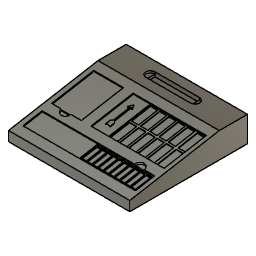
mme_projekt (Autodesk Fusion 360 design; units mm, degrees)
Autodesk Fusion 360 part; units mm, degrees
note: some values were not read from the file. Set by a fixed rule: which sketch regions a step uses.
sketch "Base" plane through (0, 0, 0) normal (1, 0, 0) x (0, 1, 0)
  line L0 (0, 0) -> (0, 20)
  line L1 (0, 20) -> (184.2, 20)
  line L2 (184.2, 20) -> (184.2, 0)
  line L3 (184.2, 0) -> (0, 0)
  line L4 (184.2, 20) -> (184.2, 52.4794)
  line L5 (184.2, 52.4794) -> (0, 20)
  line L6 (184.2, 52.4794) -> (242.2, 52.4794)
  line L7 (242.2, 52.4794) -> (242.2, 0)
  line L8 (242.2, 0) -> (184.2, 0)
  dimension "d6" = 10
  dimension "d7" = 58
  dimension "d8" = 184.2
  dimension "d9" = 20
  constraint coincident L0.start L3.end
  constraint vertical L0
  constraint perpendicular L0 L1
  constraint perpendicular L1 L2
  constraint perpendicular L0 L3
  constraint perpendicular L1 L4
  constraint perpendicular L0 L6
  constraint perpendicular L1 L7
  constraint perpendicular L2 L8
  measures "d6" angle of L1 L5
  measures "d7" distance of L2.end L7.end
  measures "d8" distance of L2.end L0.start
  measures "d9" distance of L0.start L0.end
sketch "Main Indents" plane through (0, -3.4202, 19.3969) normal (0, -0.173648, 0.984808) x (1, 0, 0)
  line L0 (0, 190.5145) -> (0, 3.473)
  line L1 (0, 3.473) -> (10, 3.473)
  line L2 (10, 3.473) -> (10, 190.5145)
  line L3 (10, 190.5145) -> (0, 190.5145)
  line L4 (8, 83.473) -> (71, 83.473)
  line L5 (71, 83.473) -> (71, 171.473)
  line L6 (71, 171.473) -> (8, 171.473)
  line L7 (8, 171.473) -> (8, 83.473)
  line L8 (181, 129.5926) -> (166, 129.5926)
  line L9 (166, 169.5926) -> (166, 129.5926)
  line L10 (166, 169.5926) -> (181, 169.5926)
  line L11 (181, 169.5926) -> (181, 129.5926)
  line L12 (147, 169.5926) -> (162, 169.5926)
  line L13 (162, 169.5926) -> (162, 129.5926)
  line L14 (128, 169.5926) -> (128, 129.5926)
  line L15 (143, 129.5926) -> (128, 129.5926)
  line L16 (147, 169.5926) -> (147, 129.5926)
  line L17 (128, 169.5926) -> (143, 169.5926)
  line L18 (143, 169.5926) -> (143, 129.5926)
  line L19 (162, 129.5926) -> (147, 129.5926)
  line L20 (162, 125.5926) -> (162, 85.5926)
  line L21 (128, 125.5926) -> (143, 125.5926)
  line L22 (166, 125.5926) -> (166, 85.5926)
  line L23 (181, 85.5926) -> (166, 85.5926)
  line L24 (166, 125.5926) -> (181, 125.5926)
  line L25 (147, 125.5926) -> (162, 125.5926)
  line L26 (128, 125.5926) -> (128, 85.5926)
  line L27 (162, 85.5926) -> (147, 85.5926)
  line L28 (147, 125.5926) -> (147, 85.5926)
  line L29 (143, 125.5926) -> (143, 85.5926)
  line L30 (143, 85.5926) -> (128, 85.5926)
  line L31 (181, 125.5926) -> (181, 85.5926)
  line L32 (143, 129.5926) -> (147, 129.5926) construction
  line L33 (162, 129.5926) -> (166, 129.5926) construction
  line L34 (166, 125.5926) -> (162, 125.5926) construction
  line L35 (147, 125.5926) -> (143, 125.5926) construction
  line L36 (185, 169.5926) -> (200, 169.5926)
  line L37 (200, 169.5926) -> (200, 129.5926)
  line L38 (185, 169.5926) -> (185, 129.5926)
  line L39 (200, 129.5926) -> (185, 129.5926)
  line L40 (204, 169.5926) -> (219, 169.5926)
  line L41 (219, 169.5926) -> (219, 129.5926)
  line L42 (204, 169.5926) -> (204, 129.5926)
  line L43 (219, 129.5926) -> (204, 129.5926)
  line L44 (224.5079, 169.5926) -> (239.5079, 169.5926)
  line L45 (239.5079, 169.5926) -> (239.5079, 129.5926)
  line L46 (224.5079, 169.5926) -> (224.5079, 129.5926)
  line L47 (239.5079, 129.5926) -> (224.5079, 129.5926)
  line L48 (185, 125.5926) -> (200, 125.5926)
  line L49 (200, 125.5926) -> (200, 85.5926)
  line L50 (185, 125.5926) -> (185, 85.5926)
  line L51 (200, 85.5926) -> (185, 85.5926)
  line L52 (204, 125.5926) -> (219, 125.5926)
  line L53 (219, 125.5926) -> (219, 85.5926)
  line L54 (204, 125.5926) -> (204, 85.5926)
  line L55 (219, 85.5926) -> (204, 85.5926)
  line L56 (224.5079, 125.5926) -> (239.5079, 125.5926)
  line L57 (239.5079, 125.5926) -> (239.5079, 85.5926)
  line L58 (224.5079, 125.5926) -> (224.5079, 85.5926)
  line L59 (239.5079, 85.5926) -> (224.5079, 85.5926)
  line L60 (185, 129.5926) -> (185, 125.5926) construction
  line L61 (185, 125.5926) -> (181, 125.5926) construction
  line L62 (181, 129.5926) -> (185, 129.5926) construction
  line L63 (204, 129.5926) -> (200, 129.5926) construction
  line L64 (200, 125.5926) -> (204, 125.5926) construction
  line L65 (204, 125.5926) -> (204, 129.5926) construction
  line L66 (224.5079, 125.5926) -> (224.5079, 129.5926) construction
  line L67 (219, 129.5926) -> (224.5079, 129.5926) construction
  line L68 (224.5079, 125.5926) -> (219, 125.5926) construction
  line L69 (91, 171.473) -> (241.5079, 171.473)
  line L70 (241.5079, 171.473) -> (241.5079, 83.473)
  line L71 (241.5079, 83.473) -> (91, 83.473)
  line L72 (91, 83.473) -> (91, 171.473)
  line L73 (71, 171.473) -> (91, 171.473) construction
  line L74 (8, 63.473) -> (241.5079, 63.473)
  line L75 (241.5079, 63.473) -> (241.5079, 23.473)
  line L76 (241.5079, 23.473) -> (8, 23.473)
  line L77 (8, 23.473) -> (8, 63.473)
  line L78 (8, 83.473) -> (8, 63.473) construction
  line L79 (71, 83.473) -> (91, 83.473) construction
  line L80 (216.5079, 58.973) -> (216.5079, 27.973)
  line L81 (225.7579, 27.973) -> (225.7579, 58.973)
  line L82 (225.7579, 58.973) -> (216.5079, 58.973)
  line L83 (216.5079, 27.973) -> (225.7579, 27.973)
  line L84 (205.2579, 58.973) -> (205.2579, 27.973)
  line L85 (214.5079, 27.973) -> (214.5079, 58.973)
  line L86 (214.5079, 58.973) -> (205.2579, 58.973)
  line L87 (205.2579, 27.973) -> (214.5079, 27.973)
  line L88 (194.0079, 58.973) -> (194.0079, 27.973)
  line L89 (203.2579, 27.973) -> (203.2579, 58.973)
  line L90 (203.2579, 58.973) -> (194.0079, 58.973)
  line L91 (194.0079, 27.973) -> (203.2579, 27.973)
  line L92 (227.7579, 58.973) -> (227.7579, 27.973)
  line L93 (237.0079, 27.973) -> (237.0079, 58.973)
  line L94 (237.0079, 58.973) -> (227.7579, 58.973)
  line L95 (227.7579, 27.973) -> (237.0079, 27.973)
  line L96 (182.7579, 58.973) -> (182.7579, 27.973)
  line L97 (192.0079, 27.973) -> (192.0079, 58.973)
  line L98 (192.0079, 58.973) -> (182.7579, 58.973)
  line L99 (182.7579, 27.973) -> (192.0079, 27.973)
  line L100 (171.5079, 58.973) -> (171.5079, 27.973)
  line L101 (180.7579, 27.973) -> (180.7579, 58.973)
  line L102 (180.7579, 58.973) -> (171.5079, 58.973)
  line L103 (171.5079, 27.973) -> (180.7579, 27.973)
  line L104 (160.2579, 58.973) -> (160.2579, 27.973)
  line L105 (169.5079, 27.973) -> (169.5079, 58.973)
  line L106 (169.5079, 58.973) -> (160.2579, 58.973)
  line L107 (160.2579, 27.973) -> (169.5079, 27.973)
  line L108 (149.0079, 58.973) -> (149.0079, 27.973)
  line L109 (158.2579, 27.973) -> (158.2579, 58.973)
  line L110 (158.2579, 58.973) -> (149.0079, 58.973)
  line L111 (149.0079, 27.973) -> (158.2579, 27.973)
  line L112 (137.7579, 58.973) -> (137.7579, 27.973)
  line L113 (147.0079, 27.973) -> (147.0079, 58.973)
  line L114 (147.0079, 58.973) -> (137.7579, 58.973)
  line L115 (137.7579, 27.973) -> (147.0079, 27.973)
  line L116 (126.5079, 58.973) -> (126.5079, 27.973)
  line L117 (135.7579, 27.973) -> (135.7579, 58.973)
  line L118 (135.7579, 58.973) -> (126.5079, 58.973)
  line L119 (126.5079, 27.973) -> (135.7579, 27.973)
  line L120 (227.7579, 58.973) -> (225.7579, 58.973) construction
  line L121 (216.5079, 58.973) -> (214.5079, 58.973) construction
  line L122 (205.2579, 58.973) -> (203.2579, 58.973) construction
  line L123 (194.0079, 58.973) -> (192.0079, 58.973) construction
  line L124 (182.7579, 58.973) -> (180.7579, 58.973) construction
  line L125 (171.5079, 58.973) -> (169.5079, 58.973) construction
  line L126 (160.2579, 58.973) -> (158.2579, 58.973) construction
  line L127 (149.0079, 58.973) -> (147.0079, 58.973) construction
  line L128 (137.7579, 58.973) -> (135.7579, 58.973) construction
  line L129 (216.5079, 27.973) -> (214.5079, 27.973) construction
  line L130 (205.2579, 27.973) -> (203.2579, 27.973) construction
  line L131 (194.0079, 27.973) -> (192.0079, 27.973) construction
  line L132 (182.7579, 27.973) -> (180.7579, 27.973) construction
  line L133 (171.5079, 27.973) -> (169.5079, 27.973) construction
  line L134 (160.2579, 27.973) -> (158.2579, 27.973) construction
  line L135 (149.0079, 27.973) -> (147.0079, 27.973) construction
  line L136 (137.7579, 27.973) -> (135.7579, 27.973) construction
  line L137 (227.7579, 27.973) -> (225.7579, 27.973) construction
  line L138 (124.5079, 60.973) -> (124.5079, 25.973)
  line L139 (239.0079, 60.973) -> (239.0079, 25.973)
  line L140 (237.0079, 58.973) -> (239.0079, 58.973) construction
  line L141 (237.0079, 27.973) -> (239.0079, 27.973) construction
  line L142 (126.5079, 58.973) -> (124.5079, 58.973) construction
  line L143 (126.5079, 27.973) -> (124.5079, 27.973) construction
  line L144 (241.5079, 83.473) -> (241.5079, 63.473) construction
  line L145 (126, 171.473) -> (126, 83.473)
  line L146 (128, 129.5926) -> (128, 125.5926) construction
  line L147 (124.5079, 60.973) -> (239.0079, 60.973)
  line L148 (239.0079, 25.973) -> (124.5079, 25.973)
  arc A0 (29.5, 83.473) -> (49.5, 83.473) centre (39.5, 83.473) ccw
  line L149 (39.5, 171.473) -> (39.5, 83.473)
  line L150 (8, 43.473) -> (241.5079, 43.473)
  line L151 (107.5, 113.6221) -> (107.5, 148.6221)
  line L152 (107.5, 148.6221) -> (103.5, 146.3127)
  line L153 (103.5, 146.3127) -> (108.5, 154.973)
  line L154 (108.5, 154.973) -> (113.5, 146.3127)
  line L155 (113.5, 146.3127) -> (109.5, 148.6221)
  line L156 (109.5, 148.6221) -> (109.5, 113.6221)
  line L157 (109.5, 113.6221) -> (113.0355, 110.0866)
  line L158 (113.0355, 110.0866) -> (113.0355, 100.0866)
  line L159 (113.0355, 100.0866) -> (109.5, 102.1624)
  line L160 (109.5, 102.1624) -> (107.5, 102.1624)
  line L161 (107.5, 102.1624) -> (103.9645, 99.973)
  line L162 (103.9645, 99.973) -> (103.9645, 110.0866)
  line L163 (103.9645, 110.0866) -> (107.5, 113.6221)
  line L164 (107.5, 148.6221) -> (109.5, 148.6221) construction
  line L165 (107.5, 113.6221) -> (107.5, 102.1624) construction
  line L166 (109.5, 113.6221) -> (109.5, 102.1624) construction
  line L167 (107.5, 113.6221) -> (109.5, 113.6221) construction
  line L168 (103.9645, 99.973) -> (103.9645, 83.473) construction
  line L169 (108.5, 154.973) -> (108.5, 171.473) construction
  line L170 (126, 154.973) -> (91, 154.973) construction
  arc A1 (220.0079, 63.473) -> (200.0079, 63.473) centre (210.0079, 63.473) ccw
  dimension "d12" = 88
  dimension "d13" = 63
  dimension "d16" = 40
  dimension "d17" = 15
  dimension "d18" = 40
  dimension "d19" = 15
  dimension "d20" = 40
  dimension "d21" = 15
  dimension "d24" = 40
  dimension "d25" = 15
  dimension "d26" = 40
  dimension "d27" = 15
  dimension "d28" = 40
  dimension "d29" = 15
  dimension "d31" = 4
  dimension "d32" = 4
  dimension "d33" = 4
  dimension "d34" = 4
  dimension "d44" = 40
  dimension "d45" = 15
  dimension "d46" = 40
  dimension "d47" = 15
  dimension "d48" = 40
  dimension "d49" = 15
  dimension "d52" = 40
  dimension "d53" = 15
  dimension "d54" = 40
  dimension "d55" = 15
  dimension "d56" = 40
  dimension "d57" = 15
  dimension "d58" = 4
  dimension "d59" = 4
  dimension "d60" = 5.5079
  dimension "d62" = 20
  dimension "d64" = 2
  dimension "d65" = 40
  dimension "d66" = 20
  dimension "d67" = 8
  dimension "d68" = 20
  dimension "d70" = 9.25
  dimension "d71" = 9.25
  dimension "d72" = 9.25
  dimension "d73" = 9.25
  dimension "d74" = 9.25
  dimension "d75" = 9.25
  dimension "d76" = 9.25
  dimension "d77" = 9.25
  dimension "d78" = 9.25
  dimension "d79" = 9.25
  dimension "d80" = 2
  dimension "d81" = 2
  dimension "d82" = 2
  dimension "d83" = 2
  dimension "d84" = 2
  dimension "d85" = 2
  dimension "d86" = 2
  dimension "d87" = 2
  dimension "d88" = 2
  dimension "d89" = 2
  dimension "d90" = 2
  dimension "d91" = 2
  dimension "d92" = 35
  dimension "d93" = 4
  dimension "d94" = 1.8804
  dimension "d95" = 2
  dimension "d96" = 2
  dimension "d97" = 2.5
  dimension "d98" = 2.5
  dimension "d99" = 2.5
  dimension "d100" = 10
  dimension "d136" = 60
  dimension "d137" = 60
  dimension "d138" = 10
  dimension "d139" = 10
  dimension "d140" = 135
  dimension "d141" = 135
  dimension "d142" = 5
  dimension "d143" = 5
  dimension "d144" = 10
  dimension "d146" = 2
  dimension "d147" = 16.5
  dimension "d148" = 16.5
  dimension "d149" = 35
  dimension "d202" = 10
  dimension "d203" = 21.5
  constraint horizontal L4
  constraint perpendicular L4 L5
  constraint perpendicular L5 L6
  constraint perpendicular L4 L7
  constraint vertical L9
  constraint perpendicular L9 L10
  constraint perpendicular L10 L11
  constraint perpendicular L8 L9
  constraint vertical L16
  constraint perpendicular L12 L16
  constraint perpendicular L12 L13
  constraint perpendicular L16 L19
  constraint vertical L14
  constraint perpendicular L14 L17
  constraint perpendicular L17 L18
  constraint perpendicular L14 L15
  constraint vertical L22
  constraint perpendicular L22 L24
  constraint perpendicular L24 L31
  constraint perpendicular L22 L23
  constraint vertical L26
  constraint perpendicular L21 L26
  constraint perpendicular L21 L29
  constraint perpendicular L26 L30
  constraint vertical L28
  constraint perpendicular L25 L28
  constraint perpendicular L20 L25
  constraint perpendicular L27 L28
  constraint perpendicular L18 L32
  constraint perpendicular L9 L33
  constraint vertical L38
  constraint perpendicular L36 L38
  constraint perpendicular L36 L37
  constraint perpendicular L38 L39
  constraint vertical L42
  constraint perpendicular L40 L42
  constraint perpendicular L40 L41
  constraint perpendicular L42 L43
  constraint vertical L46
  constraint perpendicular L44 L46
  constraint perpendicular L44 L45
  constraint perpendicular L46 L47
  constraint vertical L50
  constraint perpendicular L48 L50
  constraint perpendicular L48 L49
  constraint perpendicular L50 L51
  constraint vertical L54
  constraint perpendicular L52 L54
  constraint perpendicular L52 L53
  constraint perpendicular L54 L55
  constraint vertical L58
  constraint perpendicular L56 L58
  constraint perpendicular L56 L57
  constraint perpendicular L58 L59
  constraint perpendicular L38 L62
  constraint perpendicular L37 L63
  constraint perpendicular L49 L64
  constraint perpendicular L63 L65
  constraint perpendicular L46 L67
  constraint perpendicular L53 L68
  constraint perpendicular L31 L61
  constraint perpendicular L47 L66
  constraint perpendicular L69 L70
  constraint perpendicular L5 L71
  constraint perpendicular L72 L73
  constraint parallel L4 L74
  constraint perpendicular L4 L75
  constraint perpendicular L2 L76
  constraint perpendicular L74 L77
  constraint perpendicular L74 L78
  constraint perpendicular L72 L79
  constraint horizontal L82
  constraint vertical L80
  constraint horizontal L83
  constraint vertical L81
  constraint horizontal L86
  constraint vertical L84
  constraint horizontal L87
  constraint vertical L85
  constraint horizontal L90
  constraint vertical L88
  constraint horizontal L91
  constraint vertical L89
  constraint horizontal L94
  constraint vertical L92
  constraint horizontal L95
  constraint vertical L93
  constraint horizontal L98
  constraint vertical L96
  constraint horizontal L99
  constraint vertical L97
  constraint horizontal L102
  constraint vertical L100
  constraint horizontal L103
  constraint vertical L101
  constraint horizontal L106
  constraint vertical L104
  constraint horizontal L107
  constraint vertical L105
  constraint horizontal L110
  constraint vertical L108
  constraint horizontal L111
  constraint vertical L109
  constraint horizontal L114
  constraint vertical L112
  constraint horizontal L115
  constraint vertical L113
  constraint horizontal L118
  constraint vertical L116
  constraint horizontal L119
  constraint vertical L117
  constraint perpendicular L81 L120
  constraint perpendicular L85 L121
  constraint perpendicular L89 L122
  constraint perpendicular L97 L123
  constraint perpendicular L101 L124
  constraint perpendicular L105 L125
  constraint perpendicular L104 L126
  constraint perpendicular L113 L127
  constraint perpendicular L117 L128
  constraint perpendicular L85 L129
  constraint perpendicular L89 L130
  constraint perpendicular L96 L132
  constraint perpendicular L105 L133
  constraint perpendicular L113 L135
  constraint perpendicular L117 L136
  constraint perpendicular L109 L134
  constraint perpendicular L88 L131
  constraint perpendicular L81 L137
  constraint vertical L138
  constraint vertical L139
  constraint coincident L139 L140.end
  constraint perpendicular L139 L140
  constraint coincident L139 L141.end
  constraint perpendicular L139 L141
  constraint coincident L138 L142.end
  constraint perpendicular L138 L142
  constraint coincident L138 L143.end
  constraint perpendicular L138 L143
  constraint perpendicular L20 L34
  constraint perpendicular L28 L35
  constraint perpendicular L74 L144
  constraint coincident L69 L145.start
  constraint coincident L71 L145.end
  constraint perpendicular L71 L145
  constraint perpendicular L39 L60
  constraint perpendicular L21 L146
  constraint perpendicular L138 L148
  constraint perpendicular L139 L147
  constraint coincident L4 A0.start
  constraint coincident L4 A0.centre
  constraint midpoint L6 L149.start
  constraint midpoint L4 A0.centre
  constraint coincident A0.centre L149
  constraint coincident L77 L150.start
  constraint midpoint L75 L150.end
  constraint midpoint L77 L150.start
  constraint vertical L151
  constraint perpendicular L152 L154
  constraint perpendicular L153 L155
  constraint vertical L156
  constraint parallel L156 L158
  constraint perpendicular L158 L160
  constraint perpendicular L160 L162
  constraint perpendicular L151 L164
  constraint parallel L151 L165
  constraint parallel L156 L166
  constraint perpendicular L151 L167
  constraint coincident L71 L168.end
  constraint perpendicular L71 L168
  constraint coincident L69 L169.end
  constraint perpendicular L69 L169
  constraint coincident L145 L170.start
  constraint coincident L72 L170.end
  constraint perpendicular L72 L170
  constraint midpoint L153.end L170
  constraint coincident L74 A1.start
  constraint coincident L74 A1.centre
  measures "d12" distance of L4.end L5.end
  measures "d13" distance of L4.start L4.end
  measures "d16" distance of L9.start L8.end
  measures "d17" distance of L9.start L10.end
  measures "d18" distance of L12.start L16.end
  measures "d19" distance of L12.start L12.end
  measures "d20" distance of L14.end L14.start
  measures "d21" distance of L17.end L14.start
  measures "d24" distance of L22.end L22.start
  measures "d25" distance of L24.end L22.start
  measures "d26" distance of L21.start L26.end
  measures "d27" distance of L21.start L21.end
  measures "d28" distance of L27.end L25.start
  measures "d29" distance of L20.start L25.start
  measures "d31" distance of L16 L18
  measures "d32" distance of L9 L13
  measures "d33" distance of L20 L22
  measures "d34" distance of L28 L29
  measures "d44" distance of L36.start L38.end
  measures "d45" distance of L36.start L36.end
  measures "d46" distance of L40.start L42.end
  measures "d47" distance of L40.start L40.end
  measures "d48" distance of L44.start L46.end
  measures "d49" distance of L44.start L44.end
  measures "d52" distance of L48.start L50.end
  measures "d53" distance of L48.start L48.end
  measures "d54" distance of L52.start L54.end
  measures "d55" distance of L52.start L52.end
  measures "d56" distance of L56.start L58.end
  measures "d57" distance of L56.start L56.end
  measures "d58" distance of L31 L50
  measures "d59" distance of L49 L54
  measures "d60" distance of L53 L58
  measures "d62" distance of L5 L72
  measures "d64" distance of L45 L70
  measures "d65" distance of L74.end L75.end
  measures "d66" distance of L1 L76
  measures "d67" distance of L0 L77
  measures "d68" distance of L4.start L74.start
  measures "d70" distance of L93.end L92.start
  measures "d71" distance of L81.end L80.start
  measures "d72" distance of L85.end L84.start
  measures "d73" distance of L89.end L88.start
  measures "d74" distance of L97.end L96.start
  measures "d75" distance of L101.end L100.start
  measures "d76" distance of L105.end L104.start
  measures "d77" distance of L109.end L108.start
  measures "d78" distance of L113.end L112.start
  measures "d79" distance of L117.end L116.start
  measures "d80" distance of L93.end L140.end
  measures "d81" distance of L81.end L92.start
  measures "d82" distance of L80.start L85.end
  measures "d83" distance of L84.start L89.end
  measures "d84" distance of L88.start L97.end
  measures "d85" distance of L96.start L101.end
  measures "d86" distance of L100.start L105.end
  measures "d87" distance of L104.start L109.end
  measures "d88" distance of L108.start L113.end
  measures "d89" distance of L112.start L117.end
  measures "d90" distance of L116.start L142.end
  measures "d91" distance of L14 L145
  measures "d92" distance of L72 L145.start
  measures "d93" distance of L15 L21
  measures "d94" distance of L17 L69
  measures "d95" distance of L118 L147
  measures "d96" distance of L119 L148
  measures "d97" distance of L76 L148
  measures "d98" distance of L74 L147
  measures "d99" distance of L75 L139
  measures "d100" radius of A0
  measures "d136" angle of L151 L152
  measures "d137" angle of L155 L156
  measures "d138" distance of L152.end L153.end
  measures "d139" distance of L153.end L154.end
  measures "d140" angle of L151 L163
  measures "d141" angle of L156 L157
  measures "d142" distance of L156.end L157.end
  measures "d143" distance of L151.start L162.end
  measures "d144" distance of L157.end L158.end
  measures "d146" distance of L159.end L160.end
  measures "d147" distance of L153.end L169.end
  measures "d148" distance of L161.end L168.end
  measures "d149" distance of L151.start L151.end
  measures "d202" radius of A1
  measures "d203" distance of L74.end A1.start
extrude "Extrude16" add sketch "Base" along normal blind 249.5
sketch "Top Indents" plane through (0, 0, 52.4794) normal (0, 0, 1) x (-1, 0, 0)
  line L0 (0, -242.2) -> (0, -184.2)
  line L1 (0, -184.2) -> (-249.5, -184.2)
  line L2 (-249.5, -184.2) -> (-249.5, -242.2)
  line L3 (-249.5, -242.2) -> (0, -242.2)
  line L4 (-78.75, -222.7) -> (-78.75, -203.7)
  line L5 (-78.75, -222.7) -> (-170.75, -222.7)
  line L6 (-170.75, -222.7) -> (-170.75, -203.7)
  line L7 (-170.75, -203.7) -> (-78.75, -203.7)
  line L8 (-124.75, -222.7) -> (-124.75, -203.7)
  line L9 (-249.5, -213.2) -> (0, -213.2)
  line L10 (-124.75, -242.2) -> (-124.75, -184.2)
  arc A0 (-170.75, -203.7) -> (-170.75, -222.7) centre (-170.75, -213.2) ccw
  arc A1 (-78.75, -222.7) -> (-78.75, -203.7) centre (-78.75, -213.2) ccw
  dimension "d210" = 19
  dimension "d211" = 92
  constraint perpendicular L3 L4
  constraint perpendicular L4 L5
  constraint perpendicular L5 L6
  constraint perpendicular L6 L7
  constraint midpoint L5 L8.start
  constraint midpoint L7 L8.end
  constraint midpoint L2 L9.start
  constraint midpoint L0 L9.end
  constraint midpoint L3 L10.start
  constraint midpoint L1 L10.end
  constraint midpoint L8 L10
  constraint midpoint L6 A0.centre
  constraint midpoint L4 A1.centre
  measures "d210" distance of L4.start L4.end
  measures "d211" distance of L4.start L5.end
extrude "Extrude17" cut sketch "Top Indents" against normal blind 9 contours L4 L5 L8 L9 L10 | L5 L6 L8 L9 L10 | L4 L7 L8 L9 L10 | L6 L7 L8 L9 L10
extrude "Extrude18" cut sketch "Top Indents" against normal blind 4 contours L4 L9 A1 | L4 L9 A1 | L6 L9 A0 | L6 L9 A0
extrude "Extrude19" cut sketch "Main Indents" against normal blind 1 contours L8 L9 L10 L11 | L12 L13 L16 L19 | L14 L15 L17 L18 | L20 L25 L27 L28 | L21 L26 L29 L30 | L22 L23 L24 L31 | L36 L37 L38 L39 | L40 L41 L42 L43 | L44 L45 L46 L47 | L48 L49 L50 L51 | L52 L53 L54 L55 | L56 L57 L58 L59 | L69 L71 L72 L145 | L69 L70 L71 L145 | L151 L152 L153 L154 L155 L156 L157 L158 L159 L160 L161 L162 L163
extrude "Extrude20" cut sketch "Main Indents" against normal blind 2 contours L8 L9 L10 L11 | L12 L13 L16 L19 | L14 L15 L17 L18 | L20 L25 L27 L28 | L21 L26 L29 L30 | L22 L23 L24 L31 | L36 L37 L38 L39 | L40 L41 L42 L43 | L44 L45 L46 L47 | L48 L49 L50 L51 | L52 L53 L54 L55 | L56 L57 L58 L59 | L69 L71 L72 L145 | L69 L70 L71 L145
extrude "Extrude21" cut sketch "Main Indents" against normal blind 3 contours L69 L70 L71 L145
extrude "Extrude22" cut sketch "Main Indents" against normal blind 4 contours L8 L9 L10 L11 | L12 L13 L16 L19 | L14 L15 L17 L18 | L20 L25 L27 L28 | L21 L26 L29 L30 | L22 L23 L24 L31 | L36 L37 L38 L39 | L40 L41 L42 L43 | L44 L45 L46 L47 | L48 L49 L50 L51 | L52 L53 L54 L55 | L56 L57 L58 L59
extrude "Extrude23" cut sketch "Main Indents" against normal blind 2 contours L2 L4 L6 L149 | L2 L75 L76 L138 L139 L148 L150 | L4 L5 L6 L149 | L2 L74 L75 L138 L139 L147 L150
extrude "Extrude24" cut sketch "Main Indents" against normal blind 3 contours L80 L81 L83 L84 L85 L87 L88 L89 L91 L92 L93 L95 L96 L97 L99 L100 L101 L103 L104 L105 L107 L108 L109 L111 L112 L113 L115 L116 L117 L119 L138 L139 L148 L150 | L80 L81 L82 L84 L85 L86 L88 L89 L90 L92 L93 L94 L96 L97 L98 L100 L101 L102 L104 L105 L106 L108 L109 L110 L112 L113 L114 L116 L117 L118 L138 L139 L147 L150
extrude "Extrude25" cut sketch "Main Indents" against normal blind 4 contours L116 L117 L119 L150 | L116 L117 L118 L150 | L92 L93 L94 L150 | L92 L93 L95 L150 | L112 L113 L115 L150 | L112 L113 L114 L150 | L80 L81 L82 L150 | L80 L81 L83 L150 | L108 L109 L111 L150 | L108 L109 L110 L150 | L84 L85 L86 L150 | L84 L85 L87 L150 | L104 L105 L107 L150 | L104 L105 L106 L150 | L88 L89 L90 L150 | L88 L89 L91 L150 | L100 L101 L103 L150 | L100 L101 L102 L150 | L96 L97 L98 L150 | L96 L97 L99 L150
extrude "Extrude26" cut sketch "Main Indents" against normal blind 4 contours L4 A0 | L74 A1
sketch "Health Covers" plane through (0, 0, 0) normal (0, 0, 1) x (1, 0, 0)
  line L0 (-30, 0) -> (-30, 152.25)
  line L1 (-30, 152.25) -> (-69, 152.25)
  line L2 (-69, 152.25) -> (-69, 0)
  line L3 (-69, 0) -> (-30, 0)
  line L4 (-99, 141) -> (-138, 141)
  line L5 (-138, 141) -> (-138, 0)
  line L6 (-99, 0) -> (-99, 141)
  line L7 (-138, 0) -> (-99, 0)
  line L8 (-168, 129.75) -> (-207, 129.75)
  line L9 (-207, 129.75) -> (-207, 0)
  line L10 (-168, 0) -> (-168, 129.75)
  line L11 (-207, 0) -> (-168, 0)
  line L12 (0, 0) -> (-30, 0) construction
  line L13 (-69, 0) -> (-99, 0) construction
  line L14 (-138, 0) -> (-168, 0) construction
  line L15 (-58.5, 147.25) -> (-33.5, 147.25)
  line L16 (-33.5, 147.25) -> (-33.5, 137.25)
  line L17 (-33.5, 137.25) -> (-58.5, 137.25)
  line L18 (-58.5, 137.25) -> (-58.5, 147.25)
  arc A0 (-60.5, 147.25) -> (-60.5, 137.25) centre (-60.5, 142.25) ccw
  line L19 (-60.5, 147.25) -> (-60.5, 137.25)
  line L20 (-58.5, 147.25) -> (-60.5, 147.25) construction
  line L21 (-60.5, 137.25) -> (-58.5, 137.25) construction
  line L22 (-127.5, 126) -> (-127.5, 136)
  line L23 (-102.5, 126) -> (-127.5, 126)
  line L24 (-102.5, 136) -> (-102.5, 126)
  line L25 (-127.5, 136) -> (-102.5, 136)
  line L26 (-129.5, 136) -> (-129.5, 126)
  arc A1 (-129.5, 136) -> (-129.5, 126) centre (-129.5, 131) ccw
  line L27 (-196.5, 114.75) -> (-196.5, 124.75)
  line L28 (-171.5, 114.75) -> (-196.5, 114.75)
  line L29 (-171.5, 124.75) -> (-171.5, 114.75)
  line L30 (-196.5, 124.75) -> (-171.5, 124.75)
  line L31 (-198.5, 124.75) -> (-198.5, 114.75)
  arc A2 (-198.5, 124.75) -> (-198.5, 114.75) centre (-198.5, 119.75) ccw
  line L32 (-58.5, 125.25) -> (-58.5, 135.25)
  line L33 (-33.5, 125.25) -> (-58.5, 125.25)
  line L34 (-33.5, 135.25) -> (-33.5, 125.25)
  line L35 (-58.5, 135.25) -> (-33.5, 135.25)
  line L36 (-60.5, 135.25) -> (-60.5, 125.25)
  arc A3 (-60.5, 135.25) -> (-60.5, 125.25) centre (-60.5, 130.25) ccw
  line L37 (-58.5, 113.25) -> (-58.5, 123.25)
  line L38 (-33.5, 113.25) -> (-58.5, 113.25)
  line L39 (-33.5, 123.25) -> (-33.5, 113.25)
  line L40 (-58.5, 123.25) -> (-33.5, 123.25)
  line L41 (-60.5, 123.25) -> (-60.5, 113.25)
  arc A4 (-60.5, 123.25) -> (-60.5, 113.25) centre (-60.5, 118.25) ccw
  line L42 (-127.5, 114) -> (-127.5, 124)
  line L43 (-102.5, 114) -> (-127.5, 114)
  line L44 (-102.5, 124) -> (-102.5, 114)
  line L45 (-127.5, 124) -> (-102.5, 124)
  line L46 (-129.5, 124) -> (-129.5, 114)
  arc A5 (-129.5, 124) -> (-129.5, 114) centre (-129.5, 119) ccw
  line L47 (-127.5, 102) -> (-127.5, 112)
  line L48 (-102.5, 102) -> (-127.5, 102)
  line L49 (-102.5, 112) -> (-102.5, 102)
  line L50 (-127.5, 112) -> (-102.5, 112)
  line L51 (-129.5, 112) -> (-129.5, 102)
  arc A6 (-129.5, 112) -> (-129.5, 102) centre (-129.5, 107) ccw
  line L52 (-196.5, 102.75) -> (-196.5, 112.75)
  line L53 (-171.5, 102.75) -> (-196.5, 102.75)
  line L54 (-171.5, 112.75) -> (-171.5, 102.75)
  line L55 (-196.5, 112.75) -> (-171.5, 112.75)
  line L56 (-198.5, 112.75) -> (-198.5, 102.75)
  arc A7 (-198.5, 112.75) -> (-198.5, 102.75) centre (-198.5, 107.75) ccw
  line L57 (-196.5, 90.75) -> (-196.5, 100.75)
  line L58 (-171.5, 90.75) -> (-196.5, 90.75)
  line L59 (-171.5, 100.75) -> (-171.5, 90.75)
  line L60 (-196.5, 100.75) -> (-171.5, 100.75)
  line L61 (-198.5, 100.75) -> (-198.5, 90.75)
  arc A8 (-198.5, 100.75) -> (-198.5, 90.75) centre (-198.5, 95.75) ccw
  line L62 (-60.5, 135.25) -> (-58.5, 135.25) construction
  line L63 (-60.5, 125.25) -> (-58.5, 125.25) construction
  line L64 (-60.5, 123.25) -> (-58.5, 123.25) construction
  line L65 (-60.5, 113.25) -> (-58.5, 113.25) construction
  line L66 (-129.5, 124) -> (-127.5, 124) construction
  line L67 (-129.5, 114) -> (-127.5, 114) construction
  line L68 (-129.5, 112) -> (-127.5, 112) construction
  line L69 (-129.5, 102) -> (-127.5, 102) construction
  line L70 (-198.5, 100.75) -> (-196.5, 100.75) construction
  line L71 (-198.5, 90.75) -> (-196.5, 90.75) construction
  line L72 (-198.5, 102.75) -> (-196.5, 102.75) construction
  line L73 (-198.5, 112.75) -> (-196.5, 112.75) construction
  line L74 (-198.5, 124.75) -> (-196.5, 124.75) construction
  line L75 (-198.5, 114.75) -> (-196.5, 114.75) construction
  line L76 (-129.5, 136) -> (-127.5, 136) construction
  line L77 (-129.5, 126) -> (-127.5, 126) construction
  line L78 (-102.5, 126) -> (-102.5, 124) construction
  line L79 (-102.5, 114) -> (-102.5, 112) construction
  line L80 (-33.5, 137.25) -> (-33.5, 135.25) construction
  line L81 (-33.5, 125.25) -> (-33.5, 123.25) construction
  line L82 (-171.5, 114.75) -> (-171.5, 112.75) construction
  line L83 (-171.5, 102.75) -> (-171.5, 100.75) construction
  dimension "d124" = 152.25
  dimension "d125" = 141
  dimension "d126" = 129.75
  dimension "d127" = 30
  dimension "d128" = 30
  dimension "d129" = 30
  dimension "d130" = 39
  dimension "d131" = 39
  dimension "d132" = 39
  dimension "d152" = 2
  dimension "d153" = 25
  dimension "d154" = 10
  dimension "d155" = 5
  dimension "d156" = 2
  dimension "d157" = 25
  dimension "d158" = 10
  dimension "d159" = 5
  dimension "d160" = 2
  dimension "d161" = 25
  dimension "d162" = 10
  dimension "d163" = 5
  dimension "d164" = 2
  dimension "d165" = 25
  dimension "d166" = 10
  dimension "d167" = 5
  dimension "d168" = 2
  dimension "d169" = 25
  dimension "d170" = 10
  dimension "d171" = 5
  dimension "d172" = 2
  dimension "d173" = 2
  dimension "d174" = 2
  dimension "d175" = 25
  dimension "d176" = 10
  dimension "d177" = 5
  dimension "d178" = 2
  dimension "d179" = 25
  dimension "d180" = 10
  dimension "d181" = 5
  dimension "d182" = 2
  dimension "d183" = 25
  dimension "d184" = 10
  dimension "d185" = 5
  dimension "d186" = 2
  dimension "d187" = 25
  dimension "d188" = 10
  dimension "d189" = 5
  dimension "d190" = 2
  dimension "d191" = 2
  dimension "d192" = 2
  dimension "d193" = 2
  dimension "d194" = 5
  dimension "d195" = 3.5
  dimension "d196" = 3.5
  dimension "d197" = 5
  dimension "d198" = 3.5
  dimension "d199" = 5
  constraint vertical L0
  constraint perpendicular L0 L1
  constraint perpendicular L1 L2
  constraint perpendicular L0 L3
  constraint vertical L6
  constraint perpendicular L4 L6
  constraint perpendicular L4 L5
  constraint perpendicular L6 L7
  constraint vertical L10
  constraint perpendicular L8 L10
  constraint perpendicular L8 L9
  constraint perpendicular L10 L11
  constraint coincident L12.start origin
  constraint perpendicular L0 L12
  constraint perpendicular L6 L13
  constraint perpendicular L5 L14
  constraint horizontal L15
  constraint vertical L16
  constraint horizontal L17
  constraint vertical L18
  constraint perpendicular L1 L19
  constraint parallel L15 L20
  constraint parallel L17 L21
  constraint horizontal L25
  constraint vertical L24
  constraint horizontal L23
  constraint vertical L22
  constraint horizontal L30
  constraint vertical L29
  constraint horizontal L28
  constraint vertical L27
  constraint horizontal L35
  constraint vertical L34
  constraint horizontal L33
  constraint vertical L32
  constraint horizontal L40
  constraint vertical L39
  constraint horizontal L38
  constraint vertical L37
  constraint horizontal L45
  constraint vertical L44
  constraint horizontal L43
  constraint vertical L42
  constraint horizontal L50
  constraint vertical L49
  constraint horizontal L48
  constraint vertical L47
  constraint horizontal L55
  constraint vertical L54
  constraint horizontal L53
  constraint vertical L52
  constraint horizontal L60
  constraint vertical L59
  constraint horizontal L58
  constraint vertical L57
  constraint perpendicular L32 L62
  constraint perpendicular L32 L63
  constraint perpendicular L37 L64
  constraint perpendicular L37 L65
  constraint perpendicular L42 L66
  constraint perpendicular L42 L67
  constraint parallel L68 L69
  constraint perpendicular L57 L70
  constraint perpendicular L57 L71
  constraint perpendicular L52 L72
  constraint perpendicular L52 L73
  constraint perpendicular L27 L74
  constraint perpendicular L27 L75
  constraint perpendicular L26 L76
  constraint perpendicular L22 L77
  constraint parallel L50 L68
  constraint perpendicular L45 L78
  constraint perpendicular L35 L80
  constraint perpendicular L40 L81
  constraint perpendicular L55 L82
  constraint perpendicular L60 L83
  constraint parallel L49 L79
  constraint perpendicular L26 L77
  measures "d124" distance of L0.start L0.end
  measures "d125" distance of L6.start L4.start
  measures "d126" distance of L10.start L8.start
  measures "d127" distance of L12.start L0
  measures "d128" distance of L2 L6
  measures "d129" distance of L5 L10
  measures "d130" distance of L0.end L1.end
  measures "d131" distance of L4.end L4.start
  measures "d132" distance of L9 L10
  measures "d152" horizontal distance of L15.start A0.start
  measures "d153" distance of L15.start L15.end
  measures "d154" distance of L15.start L17.end
  measures "d155" radius of A0
  measures "d156" horizontal distance of L22.end L26.start
  measures "d157" distance of L22.end L24.start
  measures "d158" distance of L22.start L22.end
  measures "d159" radius of A1
  measures "d160" horizontal distance of L27.end L31.start
  measures "d161" distance of L27.end L29.start
  measures "d162" distance of L27.start L27.end
  measures "d163" radius of A2
  measures "d164" horizontal distance of L32.end L36.start
  measures "d165" distance of L32.end L34.start
  measures "d166" distance of L32.start L32.end
  measures "d167" radius of A3
  measures "d168" horizontal distance of L37.end L41.start
  measures "d169" distance of L37.end L39.start
  measures "d170" distance of L37.start L37.end
  measures "d171" radius of A4
  measures "d172" distance of L17 L35
  measures "d173" distance of L33 L40
  measures "d174" horizontal distance of L42.end L46.start
  measures "d175" distance of L42.end L44.start
  measures "d176" distance of L42.start L42.end
  measures "d177" radius of A5
  measures "d178" horizontal distance of L47.end L51.start
  measures "d179" distance of L47.end L49.start
  measures "d180" distance of L47.start L47.end
  measures "d181" radius of A6
  measures "d182" horizontal distance of L52.end L56.start
  measures "d183" distance of L52.end L54.start
  measures "d184" distance of L52.start L52.end
  measures "d185" radius of A7
  measures "d186" horizontal distance of L57.end L61.start
  measures "d187" distance of L57.end L59.start
  measures "d188" distance of L57.start L57.end
  measures "d189" radius of A8
  measures "d190" distance of L23 L45
  measures "d191" distance of L43 L50
  measures "d192" distance of L28 L55
  measures "d193" distance of L53 L60
  measures "d194" distance of L1 L15
  measures "d195" distance of L0 L16
  measures "d196" distance of L6 L24
  measures "d197" distance of L4 L25
  measures "d198" distance of L10 L29
  measures "d199" distance of L8 L30
extrude "Extrude15" [suppressed]
named bodies: "The thingy"
